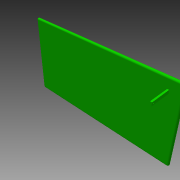
# Autodesk Inventor part: BasePlate
Saved by Autodesk Inventor 2015 (Build 190159000, 159)
## iProperties
Created: 2015-04-20
Part Number: BasePlate
Material: Generic
Document SubType Name: Modeling
Designer: WASHHSST
Density: 1 g/cm^3
Appearance: Default
Author: WASHHSST
Autodesk Inventor part; units mm, degrees
ref_plane "YZ Plane" through (0, 0, 0) normal (1, 0, 0) x (0, 1, 0)
ref_plane "XZ Plane" through (0, 0, 0) normal (0, 1, 0) x (-1, 0, 0)
ref_plane "XY Plane" through (0, 0, 0) normal (0, 0, 1) x (1, 0, 0)
sketch "Sketch1" plane through (0, 0, 0) normal (0, 0, 1) x (1, 0, 0)
  line L0 (0, 0) -> (1219.2, 0)
  line L1 (1219.2, 0) -> (1219.2, 609.6)
  line L2 (1219.2, 609.6) -> (0, 609.6)
  line L3 (0, 609.6) -> (0, 0)
  dimension "d0" = 1219.2
  dimension "d1" = 609.6
  constraints: 8 end point, 2 parallel, 1 horizontal, 1 perpendicular
  measures "d0" distance of L2.end L1.end
  measures "d1" distance of L1.end L0.end
extrude "Extrusion1" add sketch "Sketch1" along normal blind 25.4
fillet "Fillet1" radius 12.7 12 edges at (609.6, 609.6, 25.4) (609.6, 609.6, 0) (1219.2, 304.8, 25.4) (1219.2, 304.8, 0) (1219.2, 609.6, 12.7) (0, 609.6, 12.7) (0, 304.8, 25.4) (0, 304.8, 0) (609.6, 0, 0) (609.6, 0, 25.4) (0, 0, 12.7) (1219.2, 0, 12.7)
sketch "Sketch3" plane through (0, 0, 25.4) normal (0, 0, 1) x (1, 0, 0)
  line L0 (1134.1424, 536.1398) -> (1121.4424, 536.1398)
  line L1 (1121.4424, 536.1398) -> (1121.4424, 510.7398)
  line L2 (1121.4424, 510.7398) -> (1134.1424, 510.7398)
  line L3 (1134.1424, 510.7398) -> (1134.1424, 536.1398)
  point P0 (0, 0)
  dimension "d11" = 12.7
  dimension "d12" = 25.4
  constraints: 8 end point, 2 parallel, 1 horizontal, 1 perpendicular
  measures "d11" distance of L2.end L1.end
  measures "d12" distance of L1.end L0.end
extrude "Extrusion3" add sketch "Sketch3" along normal blind 152.4
sketch "Sketch4" plane through (1121.4424, 510.7398, 25.4) normal (-1, 0, 0) x (0, 0, 1)
  circle A0 centre (139.7, 12.7) radius 6.35
  line L0 (0, 25.4) -> (152.4, 25.4) projected
  line L1 (0, 0) -> (152.4, 0) projected
  line L2 (152.4, 25.4) -> (152.4, 0) projected
  point P0 (-25.4, -510.7398)
  dimension "d15" = 12.7
  dimension "d16" = 25.4
  dimension "d17" = 12.7
  dimension "d18" = 12.7
  constraints: 1 centre point
  measures "d15" diameter of A0
  measures "d16" distance between parallel lines of L0 L1
  measures "d17" distance from line of L1 A0.centre
  measures "d18" distance from line of L2 A0.centre
extrude "Extrusion4" cut sketch "Sketch4" against normal through all
body "Solid1"
